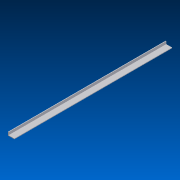
# Autodesk Inventor part: BOXC_L49_2
Saved by Autodesk Inventor 2012 (Build 160160000, 160)
## iProperties
Created: 2012-07-01
Part Number: BOXC_L49_2
Material: Default
Document SubType Name: Modeling
Designer: Hemant
Density: 1 g/cm^3
Author: Hemant
Autodesk Inventor part; units mm, degrees
ref_plane "YZ Plane" through (0, 0, 0) normal (1, 0, 0) x (0, 1, 0)
ref_plane "XZ Plane" through (0, 0, 0) normal (0, 1, 0) x (-1, 0, 0)
ref_plane "XY Plane" through (0, 0, 0) normal (0, 0, 1) x (1, 0, 0)
sketch "Sketch1" plane through (0, 0, 0) normal (0, 0, 1) x (1, 0, 0)
  line L0 (0, 0) -> (50.8, 0)
  line L1 (50.8, 0) -> (50.8, 4.7625)
  line L2 (50.8, 4.7625) -> (4.7625, 4.7625)
  line L3 (4.7625, 4.7625) -> (4.7625, 25.4)
  line L4 (4.7625, 25.4) -> (0, 25.4)
  line L5 (0, 25.4) -> (0, 0)
  dimension "d0" = 4.7625
  dimension "d1" = 4.7625
  dimension "d2" = 50.8
  dimension "d3" = 25.4
  constraints: 12 end point, 3 parallel, 2 perpendicular, 1 horizontal
  measures "d0" distance between parallel lines of L2 L0
  measures "d1" distance between parallel lines of L3 L5
  measures "d2" distance between parallel lines of L1 L5
  measures "d3" distance between parallel lines of L4 L0
extrude "Extrusion1" add sketch "Sketch1" along normal blind 1235.075
body "Solid1"
